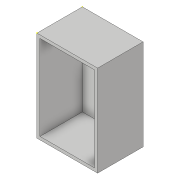
# Autodesk Inventor part: body1
Saved by Autodesk Inventor 2019 (Build 230136000, 136)
## iProperties
Created: 2020-02-12
Part Number: body1
Material: Generic
Document SubType Name: Modeling
Designer: Admin
Density: 1 g/cm^3
Appearance: Default
Author: Admin
Autodesk Inventor part; units mm, degrees
ref_plane "YZ Plane" through (0, 0, 0) normal (1, 0, 0) x (0, 1, 0)
ref_plane "XZ Plane" through (0, 0, 0) normal (0, 1, 0) x (-1, 0, 0)
sketch "Sketch1" plane through (0, 0, 0) normal (1, 0, 0) x (0, 1, 0)
  line L0 (0, 0) -> (-300, 0)
  line L1 (-300, 0) -> (-300, -150)
  line L2 (-300, -150) -> (0, -150)
  line L3 (0, -150) -> (0, 0)
  dimension "d0" = 300
  dimension "d1" = 150
  constraints: 8 end point, 2 parallel, 1 horizontal, 1 perpendicular
  measures "d0" distance of L2.end L1.end
  measures "d1" distance of L1.end L0.end
extrude "Extrusion1" add sketch "Sketch1" along normal blind 200
sketch "Sketch2" plane through (0, 0, 0) normal (-1, 0, 0) x (0, 0, 1)
  point P0 (0, 0)
sketch "Sketch3" plane through (0, -300, 0) normal (0, 0, 1) x (1, 0, 0)
  point P0 (0, 300)
sketch "Sketch4" plane through (0, -300, 0) normal (0, 0, 1) x (1, 0, 0)
  point P0 (0, 300)
sketch "Sketch5" plane through (0, -300, 0) normal (0, 0, 1) x (1, 0, 0)
  line L0 (0, 0) -> (200, 0) projected
  line L1 (0, 0) -> (190, 0)
  line L2 (190, 10) -> (190, 290)
  line L3 (190, 290) -> (0, 290)
  line L4 (0, 10) -> (0, 0)
  line L5 (-111.4723, 0) -> (-111.4723, 10)
  line L6 (10, 10) -> (190, 10)
  line L7 (0, -40.6594) -> (10, -40.6594)
  line L8 (10, 0) -> (10, 290)
  point P0 (0, 300)
  dimension "d4" = 190
  dimension "d5" = 290
  dimension "d6" = 10
  dimension "d7" = 10
  constraints: 16 end point, 3 perpendicular, 3 point on line, 2 horizontal, 2 parallel, 1 vertical
  measures "d4" distance of L3.end L2.end
  measures "d5" distance of L2.end L1.end
  measures "d6" distance of L5.start L5.end
  measures "d7" distance of L7.start L7.end
extrude "Extrusion2" cut sketch "Sketch5" against normal blind 140
ref_plane "Work Plane1" through (0, -300, -150) normal (0, 0, -1) x (-1, 0, 0)
sketch "Sketch6" plane through (0, -300, -150) normal (0, 0, -1) x (-1, 0, 0)
  point P0 (0, 300)
sketch "Sketch7" plane through (0, -300, -150) normal (0, 0, -1) x (-1, 0, 0)
  line L0 (0, 340.13) -> (-50, 340.13)
  line L1 (-50, 340.13) -> (-50, -164.6167)
  line L2 (0, 300) -> (-200, 300) projected
  line L3 (0, 300) -> (0, 225)
  line L4 (0, 0) -> (0, 300) projected
  line L5 (-50, 225) -> (-50, 275)
  line L6 (-50, 275) -> (-70, 275)
  line L7 (-70, 275) -> (-70, 175)
  line L8 (-70, 175) -> (-30, 175)
  line L9 (-30, 175) -> (-30, 275)
  line L10 (-30, 275) -> (-50, 275)
  dimension "d14" = 50
  dimension "d15" = 75
  dimension "d16" = 50
  dimension "d17" = 20
  dimension "d18" = 100
  dimension "d19" = 40
  dimension "d20" = 100
  dimension "d21" = 20
  constraints: 18 end point, 4 perpendicular, 4 point on line, 1 horizontal
  measures "d14" distance of L0.start L0.end
  measures "d15" distance of L2.start L3.end
  measures "d16" distance of L5.start L5.end
  measures "d17" distance of L5.end L6.end
  measures "d18" distance of L6.end L7.end
  measures "d19" distance of L7.end L8.end
  measures "d20" distance of L8.end L9.end
  measures "d21" distance of L9.end L5.end
extrude "Extrusion3" cut sketch "Sketch7" against normal blind 50
sketch "Sketch8" plane through (0, -300, -150) normal (0, 0, -1) x (-1, 0, 0)
  line L0 (0, 0) -> (0, 300) projected
  line L1 (0, 0) -> (0, 75)
  line L2 (-54.3985, -5.8801) -> (-4.3985, -5.8801)
  line L3 (0, 0) -> (-200, 0) projected
  line L4 (-100, 0) -> (-100, 75)
  line L5 (-54.3985, 75) -> (-34.3985, 75)
  line L6 (-34.3985, 75) -> (-34.3985, 25)
  line L7 (-34.3985, 25) -> (-74.3985, 25)
  line L8 (-74.3985, 25) -> (-74.3985, 125)
  line L9 (-74.3985, 125) -> (-34.3985, 125)
  line L10 (-34.3985, 125) -> (-34.3985, 75)
  line L11 (-10, 10) -> (-10, 290) projected
  line L12 (-200, 0) -> (-200, 300) projected
  line L13 (-200, 300) -> (-150, 300)
  line L14 (0, 300) -> (-200, 300) projected
  line L15 (-200, 300) -> (-200, 225)
  line L16 (-150, 225) -> (-170, 225)
  line L17 (-170, 225) -> (-170, 175)
  line L18 (-170, 175) -> (-130, 175)
  line L19 (-130, 175) -> (-130, 275)
  line L20 (-130, 275) -> (-170, 275)
  line L21 (-170, 275) -> (-170, 225)
  line L22 (-200, 0) -> (-200, 110.9429)
  line L23 (-200, 0) -> (-200, 75)
  line L24 (-200, 0) -> (-150, 0)
  line L25 (-150, 75) -> (-130, 75)
  line L26 (-130, 75) -> (-130, 25)
  line L27 (-130, 25) -> (-170, 25)
  line L28 (-170, 25) -> (-170, 125)
  line L29 (-170, 125) -> (-130, 125)
  line L30 (-130, 125) -> (-130, 75)
  dimension "d24" = 75
  dimension "d25" = 50
  dimension "d26" = 75
  dimension "d27" = 20
  dimension "d28" = 50
  dimension "d29" = 40
  dimension "d30" = 100
  dimension "d31" = 40
  dimension "d32" = 50
  dimension "d33" = 50
  dimension "d34" = 75
  dimension "d35" = 20
  dimension "d36" = 50
  dimension "d37" = 40
  dimension "d38" = 100
  dimension "d39" = 40
  dimension "d40" = 50
  dimension "d41" = 75
  dimension "d42" = 50
  dimension "d43" = 20
  dimension "d44" = 50
  dimension "d45" = 40
  dimension "d46" = 100
  dimension "d47" = 40
  dimension "d48" = 50
  constraints: 52 end point, 9 perpendicular, 8 point on line, 5 horizontal, 1 midpoint, 1 parallel, 1 vertical
  measures "d24" distance of L0.start L1.end
  measures "d25" distance of L2.start L2.end
  measures "d26" distance of L4.start L4.end
  measures "d27" distance of L5.start L5.end
  measures "d28" distance of L5.end L6.end
  measures "d29" distance of L6.end L7.end
  measures "d30" distance of L7.end L8.end
  measures "d31" distance of L8.end L9.end
  measures "d32" distance of L9.end L5.end
  measures "d33" distance of L12.end L13.end
  measures "d34" distance of L12.end L15.end
  measures "d35" distance of L16.start L16.end
  measures "d36" distance of L16.end L17.end
  measures "d37" distance of L17.end L18.end
  measures "d38" distance of L18.end L19.end
  measures "d39" distance of L19.end L20.end
  measures "d40" distance of L20.end L16.end
  measures "d41" distance of L3.end L23.end
  measures "d42" distance of L3.end L24.end
  measures "d43" distance of L25.start L25.end
  measures "d44" distance of L25.end L26.end
  measures "d45" distance of L26.end L27.end
  measures "d46" distance of L27.end L28.end
  measures "d47" distance of L28.end L29.end
  measures "d48" distance of L29.end L25.end
extrude "Extrusion4" cut sketch "Sketch8" against normal blind 50 contours L6 L7 L8 L9 L10 | L21 L20 L19 L18 L17 | L26 L27 L28 L29 L30
sketch "Sketch9" plane through (0, -300, -150) normal (0, 0, -1) x (-1, 0, 0)
  point P0 (0, 300)
sketch "Sketch14" plane through (0, -300, -150) normal (0, 0, -1) x (-1, 0, 0)
  line L0 (-30, 275) -> (-30, 175) projected
  line L1 (-70, 275) -> (-30, 275) projected
  line L2 (-30, 275) -> (-70, 275)
  line L3 (-70, 275) -> (-70, 175)
  line L4 (-30, 175) -> (-70, 175) projected
  line L5 (-70, 175) -> (-30, 175)
  line L6 (-30, 175) -> (-30, 275)
  line L7 (-130, 275) -> (-170, 275) projected
  line L8 (-130, 275) -> (-170, 275)
  line L9 (-170, 275) -> (-170, 175) projected
  line L10 (-170, 275) -> (-170, 175)
  line L11 (-130, 275) -> (-130, 175) projected
  line L12 (-170, 175) -> (-130, 175)
  line L13 (-130, 175) -> (-130, 275)
  line L14 (-34.3985, 25) -> (-34.3985, 125) projected
  line L15 (-74.3985, 25) -> (-74.3985, 125) projected
  line L16 (-34.3985, 125) -> (-74.3985, 125)
  line L17 (-74.3985, 125) -> (-74.3985, 25)
  line L18 (-34.3985, 25) -> (-74.3985, 25) projected
  line L19 (-74.3985, 25) -> (-34.3985, 25)
  line L20 (-34.3985, 25) -> (-34.3985, 125)
  line L21 (-130, 125) -> (-170, 125) projected
  line L22 (-130, 125) -> (-170, 125)
  line L23 (-130, 25) -> (-170, 25) projected
  line L24 (-170, 125) -> (-170, 25)
  line L25 (-170, 25) -> (-130, 25)
  line L26 (-130, 25) -> (-130, 125)
  point P0 (0, 300)
  dimension "d52" = 100
  constraints: 32 end point, 10 perpendicular, 4 collinear, 2 horizontal
  measures "d52" distance of L1.start L3.end
extrude "Extrusion5" add sketch "Sketch14" against normal blind 10
body "Solid1"
